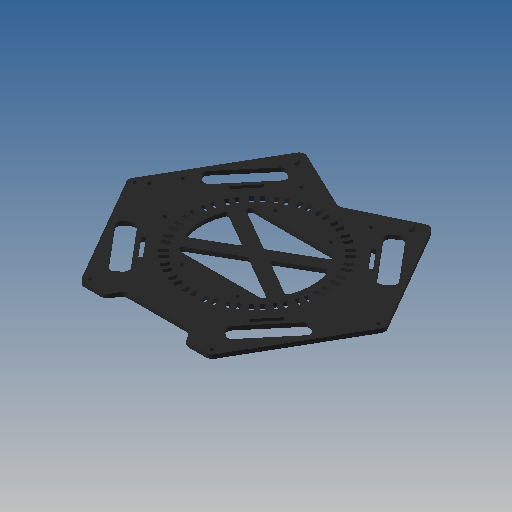
# Autodesk Inventor part: Bottom Plate
Saved by Autodesk Inventor 2017 (Build 210142000, 142)
## iProperties
Created: 2016-10-01
Part Number: Bottom Plate
Material: Polycarbonate, Clear
Document SubType Name: Modeling
Designer: James Yelland
Density: 1.2 g/cm^3
Appearance: Polycarbonate - Clear
Mass: 43.6601 g
Surface Area: 401.333 cm^2
Volume: 33.8451 cm^3
Author: James Yelland
Autodesk Inventor part; units mm, degrees
ref_plane "YZ Plane" through (0, 0, 0) normal (1, 0, 0) x (0, 1, 0)
ref_plane "XZ Plane" through (0, 0, 0) normal (0, 1, 0) x (-1, 0, 0)
ref_plane "XY Plane" through (0, 0, 0) normal (0, 0, 1) x (1, 0, 0)
sketch "Sketch1" plane through (0, 0, 0) normal (0, 1, 0) x (-1, 0, 0)
  line L0 (103.5566, -2.5) -> (54.7862, -86.9325)
  line L1 (-54.8095, -86.9325) -> (-103.5566, -2.5)
  line L2 (-103.5566, 2.5) -> (-53.9434, 88.4327)
  line L3 (53.9434, 88.4327) -> (103.5566, 2.5)
  arc A0 (48.3064, -88.9468) -> (54.7862, -86.9325) centre (50.456, -84.4325) ccw
  arc A1 (-54.8095, -86.9325) -> (-48.3297, -88.9468) centre (-50.4794, -84.4325) ccw
  arc A2 (-103.5566, 2.5) -> (-103.5566, -2.5) centre (-99.2265, 0) ccw
  arc A3 (-49.6132, 90.9327) -> (-53.9434, 88.4327) centre (-49.6132, 85.9327) ccw
  arc A4 (53.9434, 88.4327) -> (49.6132, 90.9327) centre (49.6132, 85.9327) ccw
  arc A5 (103.5566, -2.5) -> (103.5566, 2.5) centre (99.2265, 0) ccw
  circle A6 centre (49.6132, 85.9327) radius 1.6
  circle A7 centre (-49.6132, 85.9327) radius 1.6
  circle A8 centre (-99.2265, 0) radius 1.6
  circle A9 centre (99.2265, 0) radius 1.6
  line L4 (1.5, -53.75) -> (1.5, -56.75)
  line L5 (1.5, -56.75) -> (4.5, -56.75)
  line L6 (4.5, -56.75) -> (4.5, -50.75)
  line L7 (4.5, -50.75) -> (1.5, -50.75)
  line L8 (1.5, -50.75) -> (1.5, -53.75)
  line L9 (-1.5, -53.75) -> (-1.5, -56.75)
  line L10 (-1.5, -56.75) -> (-4.5, -56.75)
  line L11 (-1.5, -53.75) -> (-1.5, -53.75)
  line L12 (-1.5, -53.75) -> (-1.5, -50.75)
  line L13 (-1.5, -50.75) -> (-4.5, -50.75)
  line L14 (-4.5, -56.75) -> (-4.5, -50.75)
  line L15 (15.3604, -51.5303) -> (16.1369, -54.4281)
  line L16 (16.1369, -54.4281) -> (19.0346, -53.6516)
  line L17 (19.0346, -53.6516) -> (17.4817, -47.856)
  line L18 (17.4817, -47.856) -> (14.584, -48.6325)
  line L19 (14.584, -48.6325) -> (15.3604, -51.5303)
  line L20 (12.4626, -52.3067) -> (13.2391, -55.2045)
  line L21 (13.2391, -55.2045) -> (10.3413, -55.981)
  line L22 (12.4626, -52.3067) -> (11.6862, -49.409)
  line L23 (11.6862, -49.409) -> (8.7884, -50.1854)
  line L24 (10.3413, -55.981) -> (8.7884, -50.1854)
  line L25 (28.174, -45.7989) -> (29.674, -48.3969)
  line L26 (29.674, -48.3969) -> (32.2721, -46.8969)
  line L27 (32.2721, -46.8969) -> (29.2721, -41.7008)
  line L28 (29.2721, -41.7008) -> (26.674, -43.2008)
  line L29 (26.674, -43.2008) -> (28.174, -45.7989)
  line L30 (25.576, -47.2989) -> (27.076, -49.8969)
  line L31 (27.076, -49.8969) -> (24.4779, -51.3969)
  line L32 (25.576, -47.2989) -> (24.076, -44.7008)
  line L33 (24.076, -44.7008) -> (21.4779, -46.2008)
  line L34 (24.4779, -51.3969) -> (21.4779, -46.2008)
  line L35 (39.0676, -36.9463) -> (41.189, -39.0676)
  line L36 (41.189, -39.0676) -> (43.3103, -36.9463)
  line L37 (43.3103, -36.9463) -> (39.0676, -32.7037)
  line L38 (39.0676, -32.7037) -> (36.9463, -34.825)
  line L39 (36.9463, -34.825) -> (39.0676, -36.9463)
  line L40 (36.9463, -39.0676) -> (39.0676, -41.189)
  line L41 (39.0676, -41.189) -> (36.9463, -43.3103)
  line L42 (36.9463, -39.0676) -> (34.825, -36.9463)
  line L43 (34.825, -36.9463) -> (32.7037, -39.0676)
  line L44 (36.9463, -43.3103) -> (32.7037, -39.0676)
  line L45 (47.2989, -25.576) -> (49.8969, -27.076)
  line L46 (49.8969, -27.076) -> (51.3969, -24.4779)
  line L47 (51.3969, -24.4779) -> (46.2008, -21.4779)
  line L48 (46.2008, -21.4779) -> (44.7008, -24.076)
  line L49 (44.7008, -24.076) -> (47.2989, -25.576)
  line L50 (45.7989, -28.174) -> (48.3969, -29.674)
  line L51 (48.3969, -29.674) -> (46.8969, -32.2721)
  line L52 (45.7989, -28.174) -> (43.2008, -26.674)
  line L53 (43.2008, -26.674) -> (41.7008, -29.2721)
  line L54 (46.8969, -32.2721) -> (41.7008, -29.2721)
  line L55 (52.3067, -12.4626) -> (55.2045, -13.2391)
  line L56 (55.2045, -13.2391) -> (55.981, -10.3413)
  line L57 (55.981, -10.3413) -> (50.1854, -8.7884)
  line L58 (50.1854, -8.7884) -> (49.409, -11.6862)
  line L59 (49.409, -11.6862) -> (52.3067, -12.4626)
  line L60 (51.5303, -15.3604) -> (54.4281, -16.1369)
  line L61 (54.4281, -16.1369) -> (53.6516, -19.0346)
  line L62 (51.5303, -15.3604) -> (48.6325, -14.584)
  line L63 (48.6325, -14.584) -> (47.856, -17.4817)
  line L64 (53.6516, -19.0346) -> (47.856, -17.4817)
  line L65 (53.75, 1.5) -> (56.75, 1.5)
  line L66 (56.75, 1.5) -> (56.75, 4.5)
  line L67 (56.75, 4.5) -> (50.75, 4.5)
  line L68 (50.75, 4.5) -> (50.75, 1.5)
  line L69 (50.75, 1.5) -> (53.75, 1.5)
  line L70 (53.75, -1.5) -> (56.75, -1.5)
  line L71 (56.75, -1.5) -> (56.75, -4.5)
  line L72 (53.75, -1.5) -> (50.75, -1.5)
  line L73 (50.75, -1.5) -> (50.75, -4.5)
  line L74 (56.75, -4.5) -> (50.75, -4.5)
  line L75 (51.5303, 15.3604) -> (54.4281, 16.1369)
  line L76 (54.4281, 16.1369) -> (53.6516, 19.0346)
  line L77 (53.6516, 19.0346) -> (47.856, 17.4817)
  line L78 (47.856, 17.4817) -> (48.6325, 14.584)
  line L79 (48.6325, 14.584) -> (51.5303, 15.3604)
  line L80 (52.3067, 12.4626) -> (55.2045, 13.2391)
  line L81 (55.2045, 13.2391) -> (55.981, 10.3413)
  line L82 (52.3067, 12.4626) -> (49.409, 11.6862)
  line L83 (49.409, 11.6862) -> (50.1854, 8.7884)
  line L84 (55.981, 10.3413) -> (50.1854, 8.7884)
  line L85 (45.7989, 28.174) -> (48.3969, 29.674)
  line L86 (48.3969, 29.674) -> (46.8969, 32.2721)
  line L87 (46.8969, 32.2721) -> (41.7008, 29.2721)
  line L88 (41.7008, 29.2721) -> (43.2008, 26.674)
  line L89 (43.2008, 26.674) -> (45.7989, 28.174)
  line L90 (47.2989, 25.576) -> (49.8969, 27.076)
  line L91 (49.8969, 27.076) -> (51.3969, 24.4779)
  line L92 (47.2989, 25.576) -> (44.7008, 24.076)
  line L93 (44.7008, 24.076) -> (46.2008, 21.4779)
  line L94 (51.3969, 24.4779) -> (46.2008, 21.4779)
  line L95 (36.9463, 39.0676) -> (39.0676, 41.189)
  line L96 (39.0676, 41.189) -> (36.9463, 43.3103)
  line L97 (36.9463, 43.3103) -> (32.7037, 39.0676)
  line L98 (32.7037, 39.0676) -> (34.825, 36.9463)
  line L99 (34.825, 36.9463) -> (36.9463, 39.0676)
  line L100 (39.0676, 36.9463) -> (41.189, 39.0676)
  line L101 (41.189, 39.0676) -> (43.3103, 36.9463)
  line L102 (39.0676, 36.9463) -> (36.9463, 34.825)
  line L103 (36.9463, 34.825) -> (39.0676, 32.7037)
  line L104 (43.3103, 36.9463) -> (39.0676, 32.7037)
  line L105 (25.576, 47.2989) -> (27.076, 49.8969)
  line L106 (27.076, 49.8969) -> (24.4779, 51.3969)
  line L107 (24.4779, 51.3969) -> (21.4779, 46.2008)
  line L108 (21.4779, 46.2008) -> (24.076, 44.7008)
  line L109 (24.076, 44.7008) -> (25.576, 47.2989)
  line L110 (28.174, 45.7989) -> (29.674, 48.3969)
  line L111 (29.674, 48.3969) -> (32.2721, 46.8969)
  line L112 (28.174, 45.7989) -> (26.674, 43.2008)
  line L113 (26.674, 43.2008) -> (29.2721, 41.7008)
  line L114 (32.2721, 46.8969) -> (29.2721, 41.7008)
  line L115 (12.4626, 52.3067) -> (13.2391, 55.2045)
  line L116 (13.2391, 55.2045) -> (10.3413, 55.981)
  line L117 (10.3413, 55.981) -> (8.7884, 50.1854)
  line L118 (8.7884, 50.1854) -> (11.6862, 49.409)
  line L119 (11.6862, 49.409) -> (12.4626, 52.3067)
  line L120 (15.3604, 51.5303) -> (16.1369, 54.4281)
  line L121 (16.1369, 54.4281) -> (19.0346, 53.6516)
  line L122 (15.3604, 51.5303) -> (14.584, 48.6325)
  line L123 (14.584, 48.6325) -> (17.4817, 47.856)
  line L124 (19.0346, 53.6516) -> (17.4817, 47.856)
  line L125 (-1.5, 53.75) -> (-1.5, 56.75)
  line L126 (-1.5, 56.75) -> (-4.5, 56.75)
  line L127 (-4.5, 56.75) -> (-4.5, 50.75)
  line L128 (-4.5, 50.75) -> (-1.5, 50.75)
  line L129 (-1.5, 50.75) -> (-1.5, 53.75)
  line L130 (1.5, 53.75) -> (1.5, 56.75)
  line L131 (1.5, 56.75) -> (4.5, 56.75)
  line L132 (1.5, 53.75) -> (1.5, 50.75)
  line L133 (1.5, 50.75) -> (4.5, 50.75)
  line L134 (4.5, 56.75) -> (4.5, 50.75)
  line L135 (-15.3604, 51.5303) -> (-16.1369, 54.4281)
  line L136 (-16.1369, 54.4281) -> (-19.0346, 53.6516)
  line L137 (-19.0346, 53.6516) -> (-17.4817, 47.856)
  line L138 (-17.4817, 47.856) -> (-14.584, 48.6325)
  line L139 (-14.584, 48.6325) -> (-15.3604, 51.5303)
  line L140 (-12.4626, 52.3067) -> (-13.2391, 55.2045)
  line L141 (-13.2391, 55.2045) -> (-10.3413, 55.981)
  line L142 (-12.4626, 52.3067) -> (-11.6862, 49.409)
  line L143 (-11.6862, 49.409) -> (-8.7884, 50.1854)
  line L144 (-10.3413, 55.981) -> (-8.7884, 50.1854)
  line L145 (-28.174, 45.7989) -> (-29.674, 48.3969)
  line L146 (-29.674, 48.3969) -> (-32.2721, 46.8969)
  line L147 (-32.2721, 46.8969) -> (-29.2721, 41.7008)
  line L148 (-29.2721, 41.7008) -> (-26.674, 43.2008)
  line L149 (-26.674, 43.2008) -> (-28.174, 45.7989)
  line L150 (-25.576, 47.2989) -> (-27.076, 49.8969)
  line L151 (-27.076, 49.8969) -> (-24.4779, 51.3969)
  line L152 (-25.576, 47.2989) -> (-24.076, 44.7008)
  line L153 (-24.076, 44.7008) -> (-21.4779, 46.2008)
  line L154 (-24.4779, 51.3969) -> (-21.4779, 46.2008)
  line L155 (-39.0676, 36.9463) -> (-41.189, 39.0676)
  line L156 (-41.189, 39.0676) -> (-43.3103, 36.9463)
  line L157 (-43.3103, 36.9463) -> (-39.0676, 32.7037)
  line L158 (-39.0676, 32.7037) -> (-36.9463, 34.825)
  line L159 (-36.9463, 34.825) -> (-39.0676, 36.9463)
  line L160 (-36.9463, 39.0676) -> (-39.0676, 41.189)
  line L161 (-39.0676, 41.189) -> (-36.9463, 43.3103)
  line L162 (-36.9463, 39.0676) -> (-34.825, 36.9463)
  line L163 (-34.825, 36.9463) -> (-32.7037, 39.0676)
  line L164 (-36.9463, 43.3103) -> (-32.7037, 39.0676)
  line L165 (-47.2989, 25.576) -> (-49.8969, 27.076)
  line L166 (-49.8969, 27.076) -> (-51.3969, 24.4779)
  line L167 (-51.3969, 24.4779) -> (-46.2008, 21.4779)
  line L168 (-46.2008, 21.4779) -> (-44.7008, 24.076)
  line L169 (-44.7008, 24.076) -> (-47.2989, 25.576)
  line L170 (-45.7989, 28.174) -> (-48.3969, 29.674)
  line L171 (-48.3969, 29.674) -> (-46.8969, 32.2721)
  line L172 (-45.7989, 28.174) -> (-43.2008, 26.674)
  line L173 (-43.2008, 26.674) -> (-41.7008, 29.2721)
  line L174 (-46.8969, 32.2721) -> (-41.7008, 29.2721)
  line L175 (-52.3067, 12.4626) -> (-55.2045, 13.2391)
  line L176 (-55.2045, 13.2391) -> (-55.981, 10.3413)
  line L177 (-55.981, 10.3413) -> (-50.1854, 8.7884)
  line L178 (-50.1854, 8.7884) -> (-49.409, 11.6862)
  line L179 (-49.409, 11.6862) -> (-52.3067, 12.4626)
  line L180 (-51.5303, 15.3604) -> (-54.4281, 16.1369)
  line L181 (-54.4281, 16.1369) -> (-53.6516, 19.0346)
  line L182 (-51.5303, 15.3604) -> (-48.6325, 14.584)
  line L183 (-48.6325, 14.584) -> (-47.856, 17.4817)
  line L184 (-53.6516, 19.0346) -> (-47.856, 17.4817)
  line L185 (-53.75, -1.5) -> (-56.75, -1.5)
  line L186 (-56.75, -1.5) -> (-56.75, -4.5)
  line L187 (-56.75, -4.5) -> (-50.75, -4.5)
  line L188 (-50.75, -4.5) -> (-50.75, -1.5)
  line L189 (-50.75, -1.5) -> (-53.75, -1.5)
  line L190 (-53.75, 1.5) -> (-56.75, 1.5)
  line L191 (-56.75, 1.5) -> (-56.75, 4.5)
  line L192 (-53.75, 1.5) -> (-50.75, 1.5)
  line L193 (-50.75, 1.5) -> (-50.75, 4.5)
  line L194 (-56.75, 4.5) -> (-50.75, 4.5)
  line L195 (-51.5303, -15.3604) -> (-54.4281, -16.1369)
  line L196 (-54.4281, -16.1369) -> (-53.6516, -19.0346)
  line L197 (-53.6516, -19.0346) -> (-47.856, -17.4817)
  line L198 (-47.856, -17.4817) -> (-48.6325, -14.584)
  line L199 (-48.6325, -14.584) -> (-51.5303, -15.3604)
  line L200 (-52.3067, -12.4626) -> (-55.2045, -13.2391)
  line L201 (-55.2045, -13.2391) -> (-55.981, -10.3413)
  line L202 (-52.3067, -12.4626) -> (-49.409, -11.6862)
  line L203 (-49.409, -11.6862) -> (-50.1854, -8.7884)
  line L204 (-55.981, -10.3413) -> (-50.1854, -8.7884)
  line L205 (-45.7989, -28.174) -> (-48.3969, -29.674)
  line L206 (-48.3969, -29.674) -> (-46.8969, -32.2721)
  line L207 (-46.8969, -32.2721) -> (-41.7008, -29.2721)
  line L208 (-41.7008, -29.2721) -> (-43.2008, -26.674)
  line L209 (-43.2008, -26.674) -> (-45.7989, -28.174)
  line L210 (-47.2989, -25.576) -> (-49.8969, -27.076)
  line L211 (-49.8969, -27.076) -> (-51.3969, -24.4779)
  line L212 (-47.2989, -25.576) -> (-44.7008, -24.076)
  line L213 (-44.7008, -24.076) -> (-46.2008, -21.4779)
  line L214 (-51.3969, -24.4779) -> (-46.2008, -21.4779)
  line L215 (-36.9463, -39.0676) -> (-39.0676, -41.189)
  line L216 (-39.0676, -41.189) -> (-36.9463, -43.3103)
  line L217 (-36.9463, -43.3103) -> (-32.7037, -39.0676)
  line L218 (-32.7037, -39.0676) -> (-34.825, -36.9463)
  line L219 (-34.825, -36.9463) -> (-36.9463, -39.0676)
  line L220 (-39.0676, -36.9463) -> (-41.189, -39.0676)
  line L221 (-41.189, -39.0676) -> (-43.3103, -36.9463)
  line L222 (-39.0676, -36.9463) -> (-36.9463, -34.825)
  line L223 (-36.9463, -34.825) -> (-39.0676, -32.7037)
  line L224 (-43.3103, -36.9463) -> (-39.0676, -32.7037)
  line L225 (-25.576, -47.2989) -> (-27.076, -49.8969)
  line L226 (-27.076, -49.8969) -> (-24.4779, -51.3969)
  line L227 (-24.4779, -51.3969) -> (-21.4779, -46.2008)
  line L228 (-21.4779, -46.2008) -> (-24.076, -44.7008)
  line L229 (-24.076, -44.7008) -> (-25.576, -47.2989)
  line L230 (-28.174, -45.7989) -> (-29.674, -48.3969)
  line L231 (-29.674, -48.3969) -> (-32.2721, -46.8969)
  line L232 (-28.174, -45.7989) -> (-26.674, -43.2008)
  line L233 (-26.674, -43.2008) -> (-29.2721, -41.7008)
  line L234 (-32.2721, -46.8969) -> (-29.2721, -41.7008)
  line L235 (-12.4626, -52.3067) -> (-13.2391, -55.2045)
  line L236 (-13.2391, -55.2045) -> (-10.3413, -55.981)
  line L237 (-10.3413, -55.981) -> (-8.7884, -50.1854)
  line L238 (-8.7884, -50.1854) -> (-11.6862, -49.409)
  line L239 (-11.6862, -49.409) -> (-12.4626, -52.3067)
  line L240 (-15.3604, -51.5303) -> (-16.1369, -54.4281)
  line L241 (-16.1369, -54.4281) -> (-19.0346, -53.6516)
  line L242 (-15.3604, -51.5303) -> (-14.584, -48.6325)
  line L243 (-14.584, -48.6325) -> (-17.4817, -47.856)
  line L244 (-19.0346, -53.6516) -> (-17.4817, -47.856)
  arc A10 (50.7976, 70.0378) -> (45.1623, 70.5308) centre (47.7335, 67.4666) ccw
  line L245 (45.1623, 70.5308) -> (41.3321, 67.3169)
  arc A11 (41.3321, 67.3169) -> (40.8391, 61.6815) centre (43.9032, 64.2527) ccw
  line L246 (64.2962, 53.9509) -> (50.7976, 70.0378)
  line L247 (40.8391, 61.6815) -> (67.8361, 29.5077)
  line L248 (64.2962, 53.9509) -> (77.7947, 37.8639)
  arc A12 (77.3017, 32.2286) -> (77.7947, 37.8639) centre (74.7305, 35.2928) ccw
  line L249 (73.4714, 29.0147) -> (77.3017, 32.2286)
  arc A13 (67.8361, 29.5077) -> (73.4714, 29.0147) centre (70.9003, 32.0789) ccw
  line L250 (0, 30) -> (-31.225, 30)
  line L251 (0, 30) -> (31.225, 30)
  line L252 (0, -30) -> (-31.225, -30)
  line L253 (0, -30) -> (31.225, -30)
  arc A14 (42.1141, -15.8557) -> (42.1141, 15.8557) centre (0, 0) ccw
  arc A15 (-42.1141, 15.8558) -> (-42.1141, -15.8558) centre (0, 0) ccw
  arc A16 (34.525, 28.7563) -> (31.225, 30) centre (31.225, 25) ccw
  arc A17 (-31.225, 30) -> (-34.525, 28.7563) centre (-31.225, 25) ccw
  arc A18 (-34.525, -28.7563) -> (-31.225, -30) centre (-31.225, -25) ccw
  arc A19 (31.225, -30) -> (34.525, -28.7563) centre (31.225, -25) ccw
  circle A20 centre (22.6343, 38) radius 1.6
  circle A21 centre (-22.6343, 38) radius 1.6
  circle A22 centre (-22.6343, -38) radius 1.6
  circle A23 centre (22.6343, -38) radius 1.6
  line L254 (54.3376, 45.5946) -> (57.5515, 41.7644)
  line L255 (39.2424, -16.8831) -> (13, -1.7321)
  line L256 (39.2424, 16.8831) -> (13, 1.7321)
  line L257 (34.205, 25.5218) -> (1, 6.3509)
  line L258 (-1, 6.3509) -> (-34.205, 25.5218)
  line L259 (-39.2423, 16.8832) -> (-12.9998, 1.7321)
  line L260 (-12.9998, -1.7321) -> (-39.2423, -16.8832)
  line L261 (-34.205, -25.5218) -> (-1, -6.3509)
  line L262 (1, -6.3509) -> (34.205, -25.5218)
  arc A24 (-1, 6.3509) -> (1, 6.3509) centre (0, 8.0829) ccw
  arc A25 (-12.9998, -1.7321) -> (-12.9998, 1.7321) centre (-13.9998, 0) ccw
  arc A26 (1, -6.3509) -> (-1, -6.3509) centre (0, -8.0829) ccw
  arc A27 (13, 1.7321) -> (13, -1.7321) centre (14, 0) ccw
  arc A28 (39.2424, -16.8831) -> (42.1141, -15.8557) centre (40.2424, -15.151) ccw
  arc A29 (34.525, -28.7563) -> (34.205, -25.5218) centre (33.205, -27.2538) ccw
  arc A30 (-42.1141, -15.8558) -> (-39.2423, -16.8832) centre (-40.2423, -15.1511) ccw
  arc A31 (-34.205, -25.5218) -> (-34.525, -28.7563) centre (-33.205, -27.2538) ccw
  arc A32 (-39.2423, 16.8832) -> (-42.1141, 15.8558) centre (-40.2423, 15.1511) ccw
  arc A33 (-34.525, 28.7563) -> (-34.205, 25.5218) centre (-33.205, 27.2538) ccw
  arc A34 (42.1141, 15.8557) -> (39.2424, 16.8831) centre (40.2424, 15.151) ccw
  arc A35 (34.205, 25.5218) -> (34.525, 28.7563) centre (33.205, 27.2538) ccw
  line L263 (49.7796, 41.77) -> (43.3517, 49.4305)
  line L264 (43.3517, 49.4305) -> (45.6499, 51.3589)
  line L265 (45.6499, 51.3589) -> (58.5056, 36.038)
  line L266 (58.5056, 36.038) -> (56.2075, 34.1096)
  line L267 (56.2075, 34.1096) -> (49.7796, 41.77)
  arc A36 (73.4714, -29.0147) -> (67.8361, -29.5077) centre (70.9003, -32.0789) ccw
  arc A37 (77.7947, -37.8639) -> (77.3017, -32.2286) centre (74.7305, -35.2928) ccw
  line L268 (73.4714, -29.0147) -> (77.3017, -32.2286)
  arc A38 (45.1623, -70.5308) -> (50.7976, -70.0378) centre (47.7335, -67.4666) ccw
  line L269 (45.1623, -70.5308) -> (41.3321, -67.3169)
  arc A39 (40.8391, -61.6815) -> (41.3321, -67.3169) centre (43.9032, -64.2527) ccw
  line L270 (64.2962, -53.9509) -> (50.7976, -70.0378)
  line L271 (64.2962, -53.9509) -> (77.7947, -37.8639)
  line L272 (40.8391, -61.6815) -> (67.8361, -29.5077)
  line L273 (49.7796, -41.77) -> (43.3517, -49.4305)
  line L274 (43.3517, -49.4305) -> (45.6499, -51.3589)
  line L275 (45.6499, -51.3589) -> (58.5056, -36.038)
  line L276 (58.5056, -36.038) -> (56.2075, -34.1096)
  line L277 (56.2075, -34.1096) -> (49.7796, -41.77)
  arc A40 (-73.4714, 29.0147) -> (-67.8361, 29.5077) centre (-70.9003, 32.0789) ccw
  arc A41 (-77.7947, 37.8639) -> (-77.3017, 32.2286) centre (-74.7305, 35.2928) ccw
  line L278 (-73.4714, 29.0147) -> (-77.3017, 32.2286)
  arc A42 (-45.1623, 70.5308) -> (-50.7976, 70.0378) centre (-47.7335, 67.4666) ccw
  line L279 (-45.1623, 70.5308) -> (-41.3321, 67.3169)
  arc A43 (-40.8391, 61.6815) -> (-41.3321, 67.3169) centre (-43.9032, 64.2527) ccw
  line L280 (-64.2962, 53.9509) -> (-50.7976, 70.0378)
  line L281 (-64.2962, 53.9509) -> (-77.7947, 37.8639)
  line L282 (-40.8391, 61.6815) -> (-67.8361, 29.5077)
  line L283 (-49.7796, 41.77) -> (-43.3517, 49.4305)
  line L284 (-43.3517, 49.4305) -> (-45.6499, 51.3589)
  line L285 (-45.6499, 51.3589) -> (-58.5056, 36.038)
  line L286 (-58.5056, 36.038) -> (-56.2075, 34.1096)
  line L287 (-56.2075, 34.1096) -> (-49.7796, 41.77)
  arc A44 (-67.8361, -29.5077) -> (-73.4714, -29.0147) centre (-70.9003, -32.0789) ccw
  line L288 (-45.6499, -51.3589) -> (-58.5056, -36.038)
  line L289 (-58.5056, -36.038) -> (-56.2075, -34.1096)
  line L290 (-40.8391, -61.6815) -> (-67.8361, -29.5077)
  line L291 (-64.2962, -53.9509) -> (-77.7947, -37.8639)
  line L292 (-73.4714, -29.0147) -> (-77.3017, -32.2286)
  arc A45 (-77.3017, -32.2286) -> (-77.7947, -37.8639) centre (-74.7305, -35.2928) ccw
  line L293 (-43.3517, -49.4305) -> (-45.6499, -51.3589)
  line L294 (-49.7796, -41.77) -> (-43.3517, -49.4305)
  arc A46 (-50.7976, -70.0378) -> (-45.1623, -70.5308) centre (-47.7335, -67.4666) ccw
  line L295 (-64.2962, -53.9509) -> (-50.7976, -70.0378)
  line L296 (-45.1623, -70.5308) -> (-41.3321, -67.3169)
  arc A47 (-41.3321, -67.3169) -> (-40.8391, -61.6815) centre (-43.9032, -64.2527) ccw
  line L297 (-56.2075, -34.1096) -> (-49.7796, -41.77)
  circle A48 centre (28.2679, -64.7457) radius 1.6
  circle A49 centre (-28.2679, -64.7457) radius 1.6
  circle A50 centre (63.1808, 11.5746) radius 1.6
  circle A51 centre (92.6257, -5.4254) radius 1.6
  circle A52 centre (82.6257, -22.7459) radius 1.6
  line L298 (103.5566, -2.5) -> (94.5534, -18.0866)
  line L299 (48.2264, -83.602) -> (48.2264, -77.602)
  line L300 (48.2264, -77.602) -> (45.2264, -77.602)
  line L301 (45.2264, -77.602) -> (45.2264, -83.602)
  line L302 (45.2264, -83.602) -> (48.2264, -83.602)
  line L303 (-48.2265, -83.602) -> (-45.2265, -83.602)
  line L304 (-45.2265, -83.602) -> (-45.2265, -77.602)
  line L305 (-45.2265, -77.602) -> (-48.2265, -77.602)
  line L306 (-48.2265, -77.602) -> (-48.2265, -83.602)
  line L307 (0, 80.9327) -> (24.1132, 80.9327)
  line L308 (28.4434, 83.4327) -> (31.3301, 88.4327)
  line L309 (0, 80.9327) -> (-24.1132, 80.9327)
  line L310 (-28.4434, 83.4327) -> (-31.3301, 88.4327)
  arc A53 (35.6603, 90.9327) -> (31.3301, 88.4327) centre (35.6603, 85.9327) ccw
  arc A54 (-31.3301, 88.4327) -> (-35.6603, 90.9327) centre (-35.6603, 85.9327) ccw
  arc A55 (24.1132, 80.9327) -> (28.4434, 83.4327) centre (24.1132, 85.9327) ccw
  arc A56 (-28.4434, 83.4327) -> (-24.1132, 80.9327) centre (-24.1132, 85.9327) ccw
  line L311 (49.6132, 90.9327) -> (35.6603, 90.9327)
  line L312 (-35.6603, 90.9327) -> (-49.6132, 90.9327)
  arc A57 (2.1402, -66.9602) -> (-2.1585, -66.9605) centre (-0.0088, -71.4748) ccw
  line L313 (48.3064, -88.9468) -> (2.1402, -66.9602)
  line L314 (-2.1585, -66.9605) -> (-48.3297, -88.9468)
  point P0 (52.4787, -90.9271)
  point P1 (-52.5, 90.9327)
  point P2 (52.5, 90.9327)
  point P3 (60, 0)
  point P4 (-60, 0)
  point P5 (-60, 0)
  point P6 (38.2679, 64.7457)
  point P7 (48.2265, 73.102)
  point P8 (70.4073, 26.4435)
  point P9 (80.3658, 34.7998)
  point P10 (60, 0)
  point P11 (-33.541, 30)
  point P12 (33.541, 30)
  point P13 (-33.541, -30)
  point P14 (33.541, -30)
  point P15 (41.2298, -18.0305)
  point P16 (41.2298, 18.0305)
  point P17 (-41.2298, 18.0306)
  point P18 (-41.2298, -18.0306)
  point P19 (70.4073, -26.4435)
  point P20 (38.2679, -64.7457)
  point P21 (-70.4073, 26.4435)
  point P22 (-80.3658, 34.7998)
  point P23 (-38.2679, 64.7457)
  point P24 (-48.2265, 73.102)
  point P25 (-70.4073, -26.4435)
  point P26 (-83.093, -27.663)
  point P27 (27, 80.9327)
  point P28 (-27, 80.9327)
  dimension "d11" = 360
  dimension "d30" = 360
  dimension "d114" = 360
  dimension "d175" = 3.2
  dimension "d177" = 3.2
  dimension "d178" = 3.2
  dimension "d185" = 6
  dimension "d186" = 27
  dimension "d187" = 120
  dimension "d188" = 27
  dimension "d189" = 120
  dimension "d190" = 5
  dimension "d191" = 5
  dimension "d219" = 5
  constraints: 630 end point, 98 point on circle, 65 point on line, 58 centre point, 6 tangent, 5 equal length, 4 coincident, 2 equal radius, 2 horizontal, 2 perpendicular, 1 midpoint, 1 vertical, 1 other
  measures "d175" diameter of A50
  measures "d177" diameter of A51
  measures "d178" diameter of A52
  measures "d185" distance of L304.end L303.end
  measures "d186" distance of L309.start point (27, 80.933)
  measures "d187" angle of L308 L307
  measures "d188" distance of L309.start point (-27, 80.933)
  measures "d189" angle of L309 L310
  measures "d190" radius of A53
  measures "d191" radius of A55
  measures "d219" radius of A57
extrude "Extrusion1" add sketch "Sketch1" along normal blind 3.2
body "Solid1"
